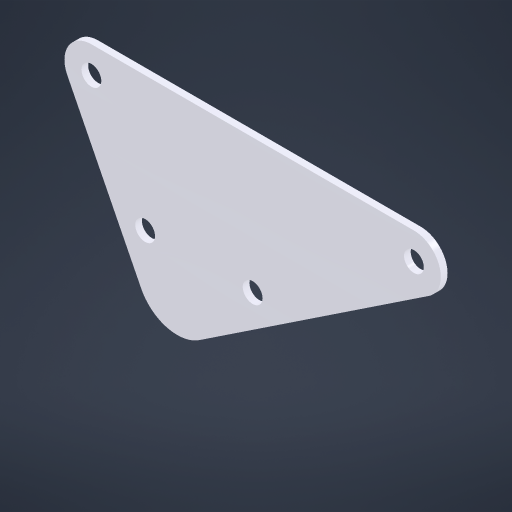
# Autodesk Inventor part: sleds
Saved by Autodesk Inventor 2024 (Build 280153000, 153)
## iProperties
Created: 2023-05-11
Part Number: sleds
Material: Polycarbonate, Clear
Document SubType Name: Sheet Metal
Designer: reima
Density: 1.2 g/cm^3
Appearance: Cool White
Sheet Metal Rule: Default_mm
Author: reima
Autodesk Inventor part; units mm, degrees
ref_plane "YZ Plane" through (0, 0, 0) normal (1, 0, 0) x (0, 1, 0)
ref_plane "XZ Plane" through (0, 0, 0) normal (0, 1, 0) x (-1, 0, 0)
ref_plane "XY Plane" through (0, 0, 0) normal (0, 0, 1) x (1, 0, 0)
sketch "Sketch12" plane through (0, 0, 0) normal (0, 0, 1) x (1, 0, 0)
  circle A0 centre (0, 0) radius 2.3368
  circle A1 centre (25.4, 0) radius 2.3368
  line L0 (-10.8766, 25.4) -> (39.9234, 25.4) construction
  circle A2 centre (-12.7, 25.4) radius 2.3368
  circle A3 centre (63.5, 25.4) radius 2.3368
  circle A4 centre (63.5, 25.4) radius 6.35
  circle A5 centre (-12.7, 25.4) radius 6.35
  circle A6 centre (0, 0) radius 6.35
  circle A7 centre (25.4, 0) radius 6.35
  line L1 (-12.7, 31.75) -> (63.5, 31.75)
  line L2 (67.0223, 20.1165) -> (12.8649, -15.9885)
  line L3 (-18.3796, 22.5602) -> (-0.9381, -12.3229)
  arc A8 (-0.9381, -12.3229) -> (12.8649, -15.9885) centre (7.5814, -8.0632) ccw
  dimension "d84" = 4.6736
  dimension "d85" = 4.6736
  dimension "d86" = 25.4
  dimension "d87" = 0
  dimension "d88" = 50.8
  dimension "d89" = 25.4
  dimension "d90" = 4.6736
  dimension "d91" = 12.7
  dimension "d92" = 4.6736
  dimension "d93" = 38.1
  dimension "d94" = 12.7
  dimension "d95" = 12.7
  dimension "d96" = 12.7
  dimension "d97" = 12.7
  dimension "d98" = 9.525
  measures "d84" diameter of A0
  measures "d85" diameter of A1
  measures "d86" distance of point (0, 0) A1.centre
  measures "d87" vertical distance of point (0, 0) A1.centre
  measures "d88" distance of L0.start L0.end
  measures "d89" distance from line of point (0, 0) L0
  measures "d90" diameter of A2
  measures "d91" horizontal distance of point (0, 0) A2.centre
  measures "d92" diameter of A3
  measures "d93" horizontal distance of A3.centre A1.centre
  measures "d94" diameter of A5
  measures "d95" diameter of A6
  measures "d96" diameter of A7
  measures "d97" diameter of A4
  measures "d98" radius of A8
extrude "Plate9" add sketch "Sketch12" along normal blind 1.5875 contours A4 | A6 | A7 | A4 L2 A8 L3 A5 L1 | A5
equation "\"d99\" = Thickness"
equation "\"BendRadius\" = Thickness"
equation "\"BendReliefWidth\" = Thickness"
equation "\"BendReliefDepth\" = 0.5 * Thickness"
equation "\"CornerReliefSize\" = 4 * Thickness"
equation "\"MinimumRemnant\" = 2 * Thickness"
equation "\"TransitionRadius\" = BendRadius"
equation "\"JacobiRadiusSize\" = BendRadius"
equation "\"GapSize\" = Thickness"
equation "\"Thickness\" = 1.5875"
body "Solid4"
